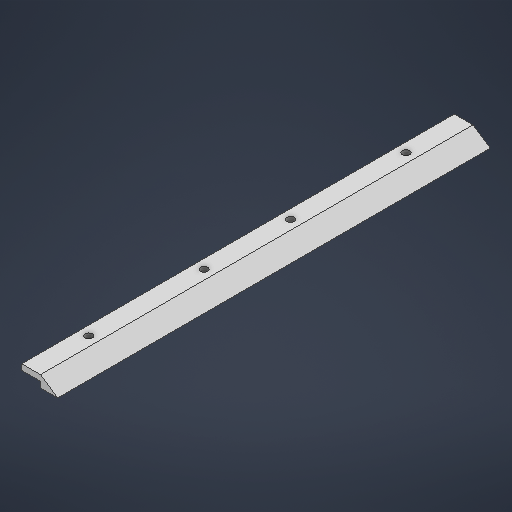
# Autodesk Inventor part: pługmoj
Saved by Autodesk Inventor 2026.2 (Build 302298010, 298A)
## iProperties
Created: 2026-05-09
Part Number: pługmoj
Material: Ogólny
Document SubType Name: Modeling
Designer: karol
Density: 1 g/cm^3
Appearance: Domyślna
Author: karol
Autodesk Inventor part; units mm, degrees
ref_plane "YZ Plane" through (0, 0, 0) normal (1, 0, 0) x (0, 1, 0)
ref_plane "XZ Plane" through (0, 0, 0) normal (0, 1, 0) x (-1, 0, 0)
ref_plane "XY Plane" through (0, 0, 0) normal (0, 0, 1) x (1, 0, 0)
sketch "Szkic1" plane through (0, 0, 0) normal (0, 1, 0) x (-1, 0, 0)
  line L0 (0, 0) -> (6.5, 0)
  line L1 (6.5, 0) -> (6.5, -150)
  line L2 (6.5, -150) -> (0, -150)
  line L3 (0, -150) -> (0, 0)
  dimension "d0" = 6.5
  dimension "d1" = 150
  constraints: 8 end point, 2 parallel, 1 horizontal, 1 perpendicular
  measures "d0" distance of L1.end L2.end
  measures "d1" distance of L0.end L1.end
extrude "Wyciągnięcie proste1" add sketch "Szkic1" along normal blind 2
sketch "Szkic2" plane through (0, 2, 0) normal (0, 1, 0) x (1, 0, 0)
  circle A0 centre (-3.25, 20) radius 1.25
  circle A1 centre (-3.25, 60) radius 1.25
  circle A2 centre (-3.25, 130) radius 1.25
  circle A3 centre (-3.25, 90) radius 1.25
  line L0 (-6.5, 0) -> (0, 0) projected
  line L1 (-6.5, 150) -> (-6.5, 0) projected
  line L2 (0, 150) -> (-6.5, 150) projected
  dimension "d4" = 20
  dimension "d5" = 3.25
  dimension "d6" = 3.25
  dimension "d7" = 60
  dimension "d8" = 60
  dimension "d9" = 20
  dimension "d10" = 3.25
  dimension "d11" = 3.25
  dimension "d12" = 2.5
  dimension "d13" = 2.5
  dimension "d14" = 2.5
  dimension "d15" = 2.5
  constraints: 4 centre point
  measures "d4" distance from line of L0 A0.centre
  measures "d5" distance from line of L1 A0.centre
  measures "d6" distance from line of L1 A1.centre
  measures "d7" distance from line of L0 A1.centre
  measures "d8" distance from line of L2 A3.centre
  measures "d9" distance from line of L2 A2.centre
  measures "d10" distance from line of L1 A2.centre
  measures "d11" distance from line of L1 A3.centre
  measures "d12" diameter of A0
  measures "d13" diameter of A1
  measures "d14" diameter of A3
  measures "d15" diameter of A2
extrude "Wyciągnięcie proste2" cut sketch "Szkic2" against normal blind 2
thread "Gwint1" size "M3x0.5" class "6H" standard "ANSI Metric M Profile" full length
thread "Gwint2" size "M3x0.5" class "6H" standard "ANSI Metric M Profile" full length
thread "Gwint3" size "M3x0.5" class "6H" standard "ANSI Metric M Profile" full length
thread "Gwint4" size "M3x0.5" class "6H" standard "ANSI Metric M Profile" full length
sketch "Szkic8" plane through (-6.5, 0, 0) normal (0, 0, 1) x (1, 0, 0)
  line L0 (6.5, 2) -> (0, 2) projected
  line L1 (6.5, 2) -> (12.5, 2)
  line L2 (12.5, 2) -> (12.5, -2)
  line L3 (12.5, -2) -> (6.5, -2)
  line L4 (6.5, -2) -> (6.5, 2)
  line L5 (12.5, -2) -> (6.5, 2)
  point P0 (6.5, 0)
  dimension "d34" = 6
  dimension "d35" = 4
  constraints: 10 end point, 2 parallel, 1 horizontal, 1 perpendicular
  measures "d34" distance of L2.end L3.end
  measures "d35" distance of L1.end L2.end
extrude "Wyciągnięcie proste6" add sketch "Szkic8" against normal blind 150 contours L5 L3 L4
